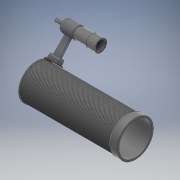
# Autodesk Inventor part: GuiderWithFinder
Saved by Autodesk Inventor 2022 (Build 260153000, 153)
## iProperties
Created: 2021-05-10
Part Number: GuiderWithFinder
Material: Generic
Document SubType Name: Modeling
Designer: Mick Veldhuis
Density: 1 g/cm^3
Appearance: Default
Author: Mick Veldhuis
Autodesk Inventor part; units mm, degrees
ref_plane "YZ Plane" through (0, 0, 0) normal (1, 0, 0) x (0, 1, 0)
sketch "Sketch3" plane through (0, 0, 0) normal (1, 0, 0) x (0, 1, 0)
  circle A0 centre (0, 0) radius 79
  constraints: 1 centre point, 1 coincident
extrude "Extrusion2" add sketch "Sketch3" along normal blind 4
sketch "Sketch4" plane through (4, 0, 0) normal (1, 0, 0) x (0, 0, -1)
  circle A0 centre (0, 0) radius 77
  circle A1 centre (0, 0) radius 73
  constraints: 2 centre point, 2 coincident
extrude "Extrusion3" add sketch "Sketch4" along normal blind 400
ref_plane "Work Plane1" through (404, 0, 0) normal (1, 0, 0) x (0, 0, -1)
sketch "Sketch5" plane through (404, 0, 0) normal (1, 0, 0) x (0, 0, -1)
  circle A0 centre (0, 0) radius 81
  circle A1 centre (0, 0) radius 73
  constraints: 2 centre point, 2 coincident
extrude "Extrusion4" add sketch "Sketch5" along normal blind 40
chamfer "Chamfer1" distance 4 angle 60 1 edges at (404, 0, 81) measured on face at (404, 0, 78.1669)
sketch "Sketch7" plane through (0, 0, 0) normal (-1, 0, 0) x (0, 0, 1)
  circle A0 centre (0, 0) radius 16
  circle A1 centre (0, 0) radius 40
  circle A2 centre (0, 0) radius 14
  constraints: 3 centre point, 2 coincident
extrude "Extrusion5" add sketch "Sketch7" along normal blind 20 contours A1
extrude "Extrusion6" add sketch "Sketch7" along normal blind 40 contours A0
fillet "Fillet1" radius 0.8 1 edges at (-40, 0, -16)
chamfer "Chamfer2" distance 8 angle 45 1 edges at (-20, 0, -40)
fillet "Fillet2" radius 1 2 edges at (444, 0, 81) (444, 0, 73)
extrude "Extrusion7" cut sketch "Sketch7" against normal through all contours A2
sketch "Sketch8" plane through (0, 0, 0) normal (-1, 0, 0) x (0, 0, 1)
  point P0 (0, 0)
sketch "Sketch9" plane through (0, 0, 0) normal (-1, 0, 0) x (0, 0, 1)
  circle A0 centre (0, 0) radius 14
  line L0 (0, 0) -> (-141.421356, 141.421356)
  line L1 (0, 0) -> (200, 0) construction
  line L2 (-50, 50) -> (-38, 62)
  line L3 (-50, 50) -> (-62, 38)
  line L4 (-38, 62) -> (-46, 70)
  line L5 (-46, 70) -> (-70, 46)
  line L6 (-70, 46) -> (-62, 38)
  dimension "d23" = 200
  dimension "d24" = 135
  constraints: 14 end point, 2 perpendicular, 2 point on line, 1 equal length, 1 horizontal
  measures "d23" distance of L0.start L0.end
  measures "d24" angle of L1 L0
extrude "Extrusion8" add sketch "Sketch9" along normal blind 6 contours L3 L6 L5 L0 | L0 L5 L4 L2
sketch "Sketch10" plane through (-6, 62, -38) normal (0, -0.7071068, 0.7071068) x (1, 0, 0)
  line L0 (6, 0) -> (6, -33.941125)
  line L1 (0, -34) -> (6, -34)
  line L2 (6, -34) -> (6, 0)
  line L3 (6, 0) -> (0, 0)
  line L4 (0, 0) -> (0, -34)
  point P0 (6, -16.970563)
  constraints: 8 end point, 2 parallel, 1 horizontal, 1 perpendicular
extrude "Extrusion9" add sketch "Sketch10" along normal blind 10
sketch "Sketch11" plane through (0, 0, 0) normal (1, 0, 0) x (0, 0, -1)
  line L0 (42.557309, 66.557309) -> (46, 70)
  line L1 (46, 70) -> (70, 46)
  line L2 (70, 46) -> (68, 44)
  line L3 (70, 46) -> (66.557309, 42.557309)
  line L4 (68, 44) -> (44, 68)
  line L5 (70, 46) -> (62, 38)
  line L6 (44, 68) -> (46, 70)
  point P0 (0, 0)
  constraints: 8 end point, 3 perpendicular, 1 point on line
extrude "Extrusion10" add sketch "Sketch11" along normal blind 50
fillet "Fillet3" radius 0.5 3 edges at (-6, 42.9081, -42.9497) (-3, 30.8873, -54.9706) (-3, 54.9289, -30.9289)
fillet "Fillet4" radius 2 1 edges at (-6, 58, -58)
fillet "Fillet5" radius 0.5 4 edges at (50, 58, -58) (50, 45, -69) (50, 56, -56) (50, 69, -45)
sketch "Sketch12" plane through (49.5, 46, -70) normal (0, 0.7071068, -0.7071068) x (-1, 0, 0)
  line L0 (4, 4) -> (50, 4)
  line L1 (50, 4) -> (50, 30)
  line L2 (50, 30) -> (4, 30)
  line L3 (4, 30) -> (4, 4)
  point P0 (49.5, 16.970563)
  constraints: 8 end point, 2 parallel, 1 horizontal, 1 perpendicular
extrude "Extrusion11" add sketch "Sketch12" along normal blind 20
sketch "Sketch13" plane through (49.5, 60.142136, -84.142136) normal (0, 0.7071068, -0.7071068) x (-1, 0, 0)
  line L0 (42, 12) -> (12, 12)
  line L1 (12, 12) -> (12, 22)
  line L2 (12, 22) -> (42, 22)
  line L3 (42, 22) -> (42, 12)
  point P0 (49.5, 16.970563)
  constraints: 8 end point, 2 parallel, 1 horizontal, 1 perpendicular
extrude "Extrusion12" add sketch "Sketch13" along normal blind 73
chamfer "Chamfer3" distance 70 angle 4 1 edges at (37.5, 123.7817, -123.7401) measured on face at (37.5, 105.397, -107.7124)
chamfer "Chamfer4" distance 8 angle 30 1 edges at (22.5, 62.9706, -81.3137) measured on face at (30.1667, 53.5425, -71.8856)
chamfer "Chamfer5" distance 8 angle 30 1 edges at (22.5, 81.3553, -62.9289) measured on face at (14.8333, 71.9272, -53.5008)
ref_plane "Work Plane3" through (7.5, 68.627417, -75.656854) normal (-1, 0, 0) x (0, -0.7071068, 0.7071068)
sketch "Sketch15" plane through (7.5, 68.627417, -75.656854) normal (-1, 0, 0) x (0, -0.7071068, 0.7071068)
  circle A0 centre (-98, 4.970563) radius 26.029437
  circle A1 centre (-98, 4.970563) radius 24.029437
  point P0 (102.024387, 4.970563)
  constraints: 2 centre point, 1 coincident
extrude "Extrusion13" add sketch "Sketch15" along normal blind 10
sketch "Sketch16" plane through (7.5, 68.627417, -75.656854) normal (1, 0, 0) x (0, -0.7071068, -0.7071068)
  circle A0 centre (-4.970563, 98) radius 26.029437
  circle A1 centre (-4.970563, 98) radius 24.029437
  point P0 (-4.970563, -102.024387)
  constraints: 2 centre point, 1 coincident
extrude "Extrusion14" add sketch "Sketch16" along normal blind 40
sketch "Sketch17" plane through (7.5, 68.627417, -75.656854) normal (-1, 0, 0) x (0, -0.7071068, 0.7071068)
  circle A0 centre (-98, 4.970563) radius 24.029437
  circle A1 centre (-98, 4.970563) radius 22.029437
  point P0 (102.024387, 4.970563)
  constraints: 2 centre point, 1 coincident
extrude "Extrusion15" add sketch "Sketch17" along normal blind 18
sketch "Sketch18" plane through (-10.5, 141.4386, -141.4386) normal (-1, 0, 0) x (0, 0, 1)
  circle A0 centre (0, 0) radius 24.029437
  point P0 (141.4386, -141.4386)
  constraints: 1 centre point
extrude "Extrusion16" add sketch "Sketch18" along normal blind 2
sketch "Sketch19" plane through (-12.5, 141.4386, -141.4386) normal (-1, 0, 0) x (0, 0, 1)
  circle A0 centre (0, 0) radius 13
  point P0 (141.4386, -141.4386)
  constraints: 1 centre point
extrude "Extrusion17" add sketch "Sketch19" along normal blind 6
sketch "Sketch20" plane through (-18.5, 141.4386, -141.4386) normal (-1, 0, 0) x (0, 0, 1)
  circle A0 centre (0, 0) radius 8
  point P0 (141.4386, -141.4386)
  dimension "d58" = 16
  constraints: 1 centre point
  measures "d58" diameter of A0
extrude "Extrusion18" add sketch "Sketch20" along normal blind 32
sketch "Sketch21" plane through (7.5, 141.4386, -141.4386) normal (1, 0, 0) x (0, 0, -1)
  circle A0 centre (0, 0) radius 22.029437
  circle A1 centre (0, 0) radius 24.029437
  point P0 (-141.4386, -141.4386)
  constraints: 2 centre point, 1 coincident
extrude "Extrusion19" add sketch "Sketch21" along normal blind 100
sketch "Sketch22" plane through (107.5, 141.4386, -141.4386) normal (1, 0, 0) x (0, 0, -1)
  circle A0 centre (0, 0) radius 8 projected
  circle A1 centre (0, 0) radius 27
  circle A2 centre (0, 0) radius 22
  point P0 (-141.4386, -141.4386)
  constraints: 2 centre point, 2 coincident
extrude "Extrusion20" add sketch "Sketch22" along normal blind 40 contours A1
fillet "Fillet6" radius 0.5 3 edges at (147.5, 141.4386, -114.4386) (107.5, 141.4386, -114.4386) (147.5, 141.4386, -119.4386)
fillet "Fillet7" radius 1 2 edges at (-18.5, 141.4386, -154.4386) (-12.5, 141.4386, -165.468)
fillet "Fillet8" radius 0.5 1 edges at (-50.5, 141.4386, -149.4386)
sketch "Sketch30" plane through (4, 0, 0) normal (1, 0, 0) x (0, 0, -1)
  line L0 (0, 0) -> (55.861436, -55.861436)
  circle A0 centre (0, 0) radius 79
  line L1 (0, 0) -> (79, 0) construction
  circle A1 centre (0, 0) radius 77
  line L2 (64.536811, -42) -> (65.981503, -43.444692)
  arc A2 (42.557309, 66.557309) -> (66.557309, 42.557309) centre (0, 0) ccw
  line L3 (64.536811, -42) -> (66.579914, -42) construction
  line L4 (42, -64.536811) -> (43.444692, -65.981503)
  line L5 (65.981503, -43.444692) -> (70, -47.463189)
  line L6 (70, -47.463189) -> (47.463189, -70)
  line L7 (47.463189, -70) -> (43.444692, -65.981503)
  arc A3 (42, -64.536811) -> (64.536811, -42) centre (0, 0) ccw
  point P0 (54.447222, -54.447222)
  dimension "d86" = 45
  dimension "d87" = 45
  constraints: 16 end point, 7 point on circle, 2 equal length, 2 horizontal, 2 perpendicular, 1 centre point, 1 parallel
  measures "d86" angle of L0 L1
  measures "d87" angle of L2 L3
extrude "Extrusion27" add sketch "Sketch30" along normal blind 400 contours A1 L2 A0 L0 | A0 L5 L6 L7
sketch "Sketch31" plane through (404, -47.463189, -70) normal (0, -0.7071068, -0.7071068) x (-1, 0, 0)
  point P0 (404, -15.935932)
sketch "Sketch32" plane through (404, -47.463189, -70) normal (0, -0.7071068, -0.7071068) x (-1, 0, 0)
  line L0 (0, 0) -> (400, 0)
  line L1 (0, 0) -> (400, 0)
  line L2 (400, 0) -> (400, -31.871864)
  line L3 (400, -31.871864) -> (0, -31.871864)
  line L4 (0, -31.871864) -> (0, 0)
  point P0 (404, -15.935932)
  constraints: 8 end point, 2 parallel, 1 horizontal, 1 perpendicular
extrude "Extrusion28" add sketch "Sketch32" along normal blind 10
sketch "Sketch33" plane through (404, -42, -64.536811) normal (0, 0.7071068, -0.7071068) x (-1, 0, 0)
  line L0 (0, 0) -> (400, 0) projected
  line L1 (8, 0) -> (392, 0)
  line L2 (392, 0) -> (392, -8)
  line L3 (392, -8) -> (8, -8)
  line L4 (8, -8) -> (8, 0)
  point P0 (404, 75.332902)
  point P1 (392, 0)
  constraints: 8 end point, 2 parallel, 1 horizontal, 1 perpendicular, 1 point on line
extrude "Extrusion29" cut sketch "Sketch33" against normal up to surface (31.871864 mm away)
sketch "Sketch34" plane through (404, -54.534257, -77.071068) normal (0, -0.7071068, -0.7071068) x (-1, 0, 0)
  point P0 (404, -15.935932)
sketch "Sketch35" plane through (404, -54.534257, -77.071068) normal (0, -0.7071068, -0.7071068) x (-1, 0, 0)
  point P0 (404, -15.935932)
  point P1 (14, -15.935932)
  point P2 (385, -15.935932)
hole "Hole1" at (19, -65.802662, -65.802662) at (390, -65.802662, -65.802662) direction (0, 0.7071068, 0.7071068) diameter 4.917 depth 9.726116 thread size "M6x1" class "6H" standard "ISO Metric profile"
sketch "Sketch36" plane through (-50.5, 141.4386, -141.4386) normal (-1, 0, 0) x (0, 0, 1)
  circle A0 centre (0, 0) radius 7
  point P0 (141.4386, -141.4386)
  constraints: 1 centre point
extrude "Extrusion30" cut sketch "Sketch36" against normal through all
body "Solid2"
